Autodesk Fusion 360 part; units mm, degrees
note: some values were not read from the file. Chosen so that the rebuilt part matches the saved one: which bodies a step acts on. Set by a fixed rule: which sketch regions a step uses.
(part 5 of 6)
sketch "Sketch100" plane through (0, 0, 40) normal (0, 0, 1) x (-1, 0, 0)
  line L0 (-66.1667, -42.5926) -> (-61.6667, -42.5926)
  line L1 (-61.6667, -42.5926) -> (-61.6667, -61.6667)
  line L2 (-61.6667, -61.6667) -> (-42.5926, -61.6667)
  line L3 (-42.5926, -61.6667) -> (-42.5926, -66.1667)
  line L4 (-42.5926, -66.1667) -> (-24.0741, -66.1667)
  line L5 (-24.0741, -66.1667) -> (-24.0741, -61.6667)
  line L6 (-24.0741, -61.6667) -> (-5, -61.6667)
  line L7 (-5, -61.6667) -> (-5, -42.5926)
  line L8 (-5, -42.5926) -> (-0.5, -42.5926)
  line L9 (-0.5, -42.5926) -> (-0.5, -24.0741)
  line L10 (-0.5, -24.0741) -> (-5, -24.0741)
  line L11 (-5, -24.0741) -> (-5, -5)
  line L12 (-5, -5) -> (-24.0741, -5)
  line L13 (-24.0741, -5) -> (-24.0741, -0.5)
  line L14 (-24.0741, -0.5) -> (-42.5926, -0.5)
  line L15 (-42.5926, -0.5) -> (-42.5926, -5)
  line L16 (-42.5926, -5) -> (-61.6667, -5)
  line L17 (-61.6667, -5) -> (-61.6667, -24.0741)
  line L18 (-61.6667, -24.0741) -> (-66.1667, -24.0741)
  line L19 (-66.1667, -24.0741) -> (-66.1667, -42.5926)
  line L20 (-20.9586, -20.9586) -> (-18.6369, -23.2802)
  line L21 (-20.9586, -20.9586) -> (-23.2802, -18.6369)
  line L22 (-18.6369, -23.2802) -> (-28.69, -33.3333)
  line L23 (-18.6369, -43.3864) -> (-28.69, -33.3333)
  line L24 (-33.3333, -37.9767) -> (-43.3864, -48.0298)
  line L25 (-33.3333, -28.69) -> (-43.3864, -18.6369)
  line L26 (-20.9586, -45.7081) -> (-23.2802, -48.0298)
  line L27 (-20.9586, -45.7081) -> (-18.6369, -43.3864)
  line L28 (-23.2802, -18.6369) -> (-33.3333, -28.69)
  line L29 (-48.0298, -43.3864) -> (-37.9767, -33.3333)
  line L30 (-45.7081, -20.9586) -> (-48.0298, -23.2802)
  line L31 (-48.0298, -23.2802) -> (-37.9767, -33.3333)
  line L32 (-43.3864, -18.6369) -> (-45.7081, -20.9586)
  line L33 (-43.3864, -48.0298) -> (-45.7081, -45.7081)
  line L34 (-45.7081, -45.7081) -> (-48.0298, -43.3864)
  line L35 (-23.2802, -48.0298) -> (-33.3333, -37.9767)
  dimension "d733" = 3.2833
  dimension "d734" = 3.2833
  dimension "d735" = 14.2173
  dimension "d736" = 14.2173
  dimension "d737" = 3.2833
  dimension "d738" = 3.2833
  dimension "d739" = 28.19
  constraint perpendicular L26 L35
  constraint perpendicular L24 L35
  constraint perpendicular L29 L34
  constraint perpendicular L23 L27
  measures "d733" distance of L26.end L26.start
  measures "d734" distance of L26.start L23.start
  measures "d735" distance of L26.end L24.start
  measures "d736" distance of L24.start L24.end
  measures "d737" distance of L33.end L24.end
  measures "d738" distance of L33.end L29.start
  measures "d739" distance of L19 L29.end
extrude "Extrude61" cut sketch "Sketch93" sketch "Sketch95" sketch "Sketch97" sketch "Sketch100" sketch "Sketch96" against normal blind 4 contours L20 L21 L22 L23 L24 L25 L26 L27 L28 L29 L30 L31 L32 L33 L34 L35 of sketch 2 contours L20 L21 L22 L23 L24 L25 L26 L27 L28 L29 L30 L31 L32 L33 L34 L35 of sketch 3 contours L20 L21 L22 L23 L24 L25 L26 L27 L28 L29 L30 L31 L32 L33 L34 L35 of sketch 4 contours L20 L21 L22 L23 L24 L25 L26 L27 L28 L29 L30 L31 L32 L33 L34 L35 of sketch 5 contours L20 L21 L22 L23 L24 L25 L26 L27 L28 L29 L30 L31 L32 L33 L34 L35 bodies 13 14 15 17 18
move_body "Align1" bodies 4 to x (-0.707107, -0.707107, 0) y (0, 0, 1) z (-0.707107, 0.707107, 0) at (170.1564, 166.6217, -160)
move_body "Align2" bodies 3 to x (0, 0, 1) y (0, 1, 0) z (-1, 0, 0) at (220, 0, -160)
move_body "Align3" bodies 1 to x (0, 0, -1) y (-1, 0, 0) z (0, 1, 0) at (228.3333, 70.7407, 40)
move_body "Align4" bodies 10 to x (1, 0, 0) y (0, 0, 1) z (0, -1, 0) at (0, 110.6667, -30.6667)
move_body "Align5" bodies 11 to x (1, 0, 0) y (0, 0, 1) z (0, -1, 0) at (0, 149.3333, -97.3333)
move_body "Align6" bodies 12 to x (1, 0, 0) y (0, 0, 1) z (0, -1, 0) at (0, 133.3333, -95.3333)
move_body "Align7" bodies 5 to x (0, 0, -1) y (0, 1, 0) z (1, 0, 0) at (62.6667, 0, 100.6667)
move_body "Align8" bodies 6 to x (0, 0, 1) y (0, 1, 0) z (-1, 0, 0) at (112, -96, -28.6667)
move_body "Align9" bodies 7 to x (0, 0, -1) y (-1, 0, 0) z (0, 1, 0) at (296, 88, 167.3333)
move_body "Align10" bodies 8 to x (0, 0, -1) y (-1, 0, 0) z (0, 1, 0) at (296, 88, 171.3333)
move_body "Align11" bodies 9 to x (0, 1, 0) y (0, 0, 1) z (1, 0, 0) at (88, 96, -28.6667)
move_body "Align12" bodies 2 to x (1, 0, 0) y (0, 0, 1) z (0, -1, 0) at (0, 24, 34)
move_body "Move1" bodies 1 to x (1, 0, 0) y (0, 1, 0) z (0, 0, 1) at (-301.8229, -79.1371, 0)
move_body "Move2" bodies 2 to x (1, 0, 0) y (0, 1, 0) z (0, 0, 1) at (-268.0592, -55.8986, 0)
move_body "Move3" bodies 3 to x (1, 0, 0) y (0, 1, 0) z (0, 0, 1) at (-506.8987, -87.6592, 0)
move_body "Move4" bodies 4 to x (0.707107, 0.707107, 0) y (-0.707107, 0.707107, 0) z (0, 0, 1) at (-289.2034, -339.6643, 0)
move_body "Move5" bodies 5 to x (1, 0, 0) y (0, 1, 0) z (0, 0, 1) at (-316.3353, -293.4677, 0)
move_body "Move6" bodies 6 to x (1, 0, 0) y (0, 1, 0) z (0, 0, 1) at (-257.8958, -196.9155, 0)
move_body "Move7" bodies 7 to x (1, 0, 0) y (0, 1, 0) z (0, 0, 1) at (-204.5381, -362.0705, 0)
move_body "Move8" bodies 8 to x (1, 0, 0) y (0, 1, 0) z (0, 0, 1) at (-203.2676, -302.3606, 0)
move_body "Move9" bodies 9 to x (1, 0, 0) y (0, 1, 0) z (0, 0, 1) at (-485.6051, -398.4452, 0)
move_body "Move10" bodies 10 to x (1, 0, 0) y (0, 1, 0) z (0, 0, 1) at (-105.1453, -228.2759, 0)
move_body "Move11" bodies 11 to x (1, 0, 0) y (0, 1, 0) z (0, 0, 1) at (-55.3396, -206.1401, 0)
move_body "Move12" bodies 12 to x (1, 0, 0) y (0, 1, 0) z (0, 0, 1) at (-264.2467, -44.2717, 0)
move_body "Move13" bodies 13 to x (1, 0, 0) y (0, 1, 0) z (0, 0, 1) at (-52.5726, -34.5873, 0)
move_body "Move14" bodies 14 to x (1, 0, 0) y (0, 1, 0) z (0, 0, 1) at (-35.9707, -35.9707, 0)
move_body "Move15" bodies 15 to x (1, 0, 0) y (0, 1, 0) z (0, 0, 1) at (-13.8349, -40.1212, 0)
move_body "Move16" bodies 16 to x (1, 0, 0) y (0, 1, 0) z (0, 0, 1) at (-38.7377, -22.1358, 0)
move_body "Move17" bodies 17 to x (1, 0, 0) y (0, 1, 0) z (0, 0, 1) at (-24.9028, -20.7524, 0)
move_body "Move18" [suppressed]
move_body "Move19" [suppressed]
move_body "Move20" [suppressed]
move_body "Move21" [suppressed]
sketch "Sketch101" plane through (0, 0, 0) normal (0, 0, 1) x (1, 0, 0)
  circle A0 centre (-33.9394, 156.9822) radius 16.4167
  line L0 (-1.1061, 166.2415) -> (-5.6061, 166.2415)
  line L1 (-5.6061, 166.2415) -> (-5.6061, 185.3156)
  line L2 (-5.6061, 185.3156) -> (-24.6802, 185.3156)
  line L3 (-24.6802, 185.3156) -> (-24.6802, 189.8156)
  line L4 (-24.6802, 189.8156) -> (-43.1987, 189.8156)
  line L5 (-43.1987, 189.8156) -> (-43.1987, 185.3156)
  line L6 (-43.1987, 185.3156) -> (-62.2728, 185.3156)
  line L7 (-62.2728, 185.3156) -> (-62.2728, 166.2415)
  line L8 (-62.2728, 166.2415) -> (-66.7728, 166.2415)
  line L9 (-66.7728, 166.2415) -> (-66.7728, 147.723)
  line L10 (-66.7728, 147.723) -> (-62.2728, 147.723)
  line L11 (-62.2728, 147.723) -> (-62.2728, 128.6489)
  line L12 (-62.2728, 128.6489) -> (-43.1987, 128.6489)
  line L13 (-43.1987, 128.6489) -> (-43.1987, 124.1489)
  line L14 (-43.1987, 124.1489) -> (-24.6802, 124.1489)
  line L15 (-24.6802, 124.1489) -> (-24.6802, 128.6489)
  line L16 (-24.6802, 128.6489) -> (-5.6061, 128.6489)
  line L17 (-5.6061, 128.6489) -> (-5.6061, 147.723)
  line L18 (-5.6061, 147.723) -> (-1.1061, 147.723)
  line L19 (-1.1061, 147.723) -> (-1.1061, 166.2415)
  circle A1 centre (-128.2759, 137.6134) radius 16.4167
  line L20 (-161.1092, 128.3541) -> (-156.6092, 128.3541)
  line L21 (-156.6092, 128.3541) -> (-156.6092, 109.28)
  line L22 (-156.6092, 109.28) -> (-137.5352, 109.28)
  line L23 (-137.5352, 109.28) -> (-137.5352, 104.78)
  line L24 (-137.5352, 104.78) -> (-119.0166, 104.78)
  line L25 (-119.0166, 104.78) -> (-119.0166, 109.28)
  line L26 (-119.0166, 109.28) -> (-99.9426, 109.28)
  line L27 (-99.9426, 109.28) -> (-99.9426, 128.3541)
  line L28 (-99.9426, 128.3541) -> (-95.4426, 128.3541)
  line L29 (-95.4426, 128.3541) -> (-95.4426, 146.8726)
  line L30 (-95.4426, 146.8726) -> (-99.9426, 146.8726)
  line L31 (-99.9426, 146.8726) -> (-99.9426, 165.9467)
  line L32 (-99.9426, 165.9467) -> (-119.0166, 165.9467)
  line L33 (-119.0166, 165.9467) -> (-119.0166, 170.4467)
  line L34 (-119.0166, 170.4467) -> (-137.5352, 170.4467)
  line L35 (-137.5352, 170.4467) -> (-137.5352, 165.9467)
  line L36 (-137.5352, 165.9467) -> (-156.6092, 165.9467)
  line L37 (-156.6092, 165.9467) -> (-156.6092, 146.8726)
  line L38 (-156.6092, 146.8726) -> (-161.1092, 146.8726)
  line L39 (-161.1092, 146.8726) -> (-161.1092, 128.3541)
  circle A2 centre (-200.4765, 134.8464) radius 16.4167
  line L40 (-167.6432, 144.1056) -> (-172.1432, 144.1056)
  line L41 (-172.1432, 144.1056) -> (-172.1432, 163.1797)
  line L42 (-172.1432, 163.1797) -> (-191.2173, 163.1797)
  line L43 (-191.2173, 163.1797) -> (-191.2173, 167.6797)
  line L44 (-191.2173, 167.6797) -> (-209.7358, 167.6797)
  line L45 (-209.7358, 167.6797) -> (-209.7358, 163.1797)
  line L46 (-209.7358, 163.1797) -> (-228.8099, 163.1797)
  line L47 (-228.8099, 163.1797) -> (-228.8099, 144.1056)
  line L48 (-228.8099, 144.1056) -> (-233.3099, 144.1056)
  line L49 (-233.3099, 144.1056) -> (-233.3099, 125.5871)
  line L50 (-233.3099, 125.5871) -> (-228.8099, 125.5871)
  line L51 (-228.8099, 125.5871) -> (-228.8099, 106.5131)
  line L52 (-228.8099, 106.5131) -> (-209.7358, 106.5131)
  line L53 (-209.7358, 106.5131) -> (-209.7358, 102.0131)
  line L54 (-209.7358, 102.0131) -> (-191.2173, 102.0131)
  line L55 (-191.2173, 102.0131) -> (-191.2173, 106.5131)
  line L56 (-191.2173, 106.5131) -> (-172.1432, 106.5131)
  line L57 (-172.1432, 106.5131) -> (-172.1432, 125.5871)
  line L58 (-172.1432, 125.5871) -> (-167.6432, 125.5871)
  line L59 (-167.6432, 125.5871) -> (-167.6432, 144.1056)
  line L60 (-326.8987, 90.1186) -> (-322.8987, 90.1186)
  line L61 (-322.8987, 90.1186) -> (-322.8987, 67.8964)
  line L62 (-322.8987, 67.8964) -> (-326.8987, 67.8964)
  line L63 (-326.8987, 67.8964) -> (-326.8987, 23.4519)
  line L64 (-326.8987, 23.4519) -> (-322.8987, 23.4519)
  line L65 (-322.8987, 23.4519) -> (-322.8987, 1.2297)
  line L66 (-322.8987, 1.2297) -> (-326.8987, 1.2297)
  line L67 (-326.8987, 1.2297) -> (-326.8987, -43.2147)
  line L68 (-326.8987, -43.2147) -> (-322.8987, -43.2147)
  line L69 (-322.8987, -43.2147) -> (-322.8987, -65.4369)
  line L70 (-322.8987, -65.4369) -> (-326.8987, -65.4369)
  line L71 (-326.8987, -65.4369) -> (-326.8987, -87.6592)
  line L72 (-326.8987, -87.6592) -> (-318.8987, -87.6592)
  line L73 (-318.8987, -87.6592) -> (-318.8987, -83.6592)
  line L74 (-318.8987, -83.6592) -> (-310.8987, -83.6592)
  line L75 (-310.8987, -83.6592) -> (-310.8987, -87.6592)
  line L76 (-310.8987, -87.6592) -> (-302.8987, -87.6592)
  line L77 (-302.8987, -87.6592) -> (-302.8987, -83.6592)
  line L78 (-302.8987, -83.6592) -> (-294.8987, -83.6592)
  line L79 (-294.8987, -83.6592) -> (-294.8987, -87.6592)
  line L80 (-294.8987, -87.6592) -> (-286.8987, -87.6592)
  line L81 (-286.8987, -87.6592) -> (-286.8987, 112.3408)
  line L82 (-286.8987, 112.3408) -> (-294.8987, 112.3408)
  line L83 (-294.8987, 112.3408) -> (-294.8987, 108.3408)
  line L84 (-294.8987, 108.3408) -> (-302.8987, 108.3408)
  line L85 (-302.8987, 108.3408) -> (-302.8987, 112.3408)
  line L86 (-302.8987, 112.3408) -> (-310.8987, 112.3408)
  line L87 (-310.8987, 112.3408) -> (-310.8987, 108.3408)
  line L88 (-310.8987, 108.3408) -> (-318.8987, 108.3408)
  line L89 (-318.8987, 108.3408) -> (-318.8987, 112.3408)
  line L90 (-318.8987, 112.3408) -> (-326.8987, 112.3408)
  line L91 (-326.8987, 112.3408) -> (-326.8987, 90.1186)
  line L92 (-314.8987, 49.6742) -> (-298.8987, 49.6742)
  line L93 (-298.8987, 49.6742) -> (-298.8987, 41.6742)
  line L94 (-298.8987, 41.6742) -> (-314.8987, 41.6742)
  line L95 (-314.8987, 41.6742) -> (-314.8987, 49.6742)
  line L96 (-314.8987, -16.9925) -> (-298.8987, -16.9925)
  line L97 (-298.8987, -16.9925) -> (-298.8987, -24.9925)
  line L98 (-298.8987, -24.9925) -> (-314.8987, -24.9925)
  line L99 (-314.8987, -24.9925) -> (-314.8987, -16.9925)
  line L100 (-86.4689, 53.0616) -> (-86.4689, 49.0616)
  line L101 (-86.4689, 49.0616) -> (-68.2467, 49.0616)
  line L102 (-68.2467, 49.0616) -> (-68.2467, 61.0616)
  line L103 (-68.2467, 61.0616) -> (-64.2467, 61.0616)
  line L104 (-64.2467, 61.0616) -> (-64.2467, 77.0616)
  line L105 (-64.2467, 77.0616) -> (-68.2467, 77.0616)
  line L106 (-68.2467, 77.0616) -> (-68.2467, 89.0616)
  line L107 (-68.2467, 89.0616) -> (-260.2467, 89.0616)
  line L108 (-260.2467, 89.0616) -> (-260.2467, 77.0616)
  line L109 (-260.2467, 77.0616) -> (-264.2467, 77.0616)
  line L110 (-264.2467, 77.0616) -> (-264.2467, 61.0616)
  line L111 (-264.2467, 61.0616) -> (-260.2467, 61.0616)
  line L112 (-260.2467, 61.0616) -> (-260.2467, 49.0616)
  line L113 (-260.2467, 49.0616) -> (-242.0244, 49.0616)
  line L114 (-242.0244, 49.0616) -> (-242.0244, 53.0616)
  line L115 (-242.0244, 53.0616) -> (-219.8022, 53.0616)
  line L116 (-219.8022, 53.0616) -> (-219.8022, 49.0616)
  line L117 (-219.8022, 49.0616) -> (-201.58, 49.0616)
  line L118 (-201.58, 49.0616) -> (-201.58, 69.0616)
  line L119 (-201.58, 69.0616) -> (-193.58, 69.0616)
  line L120 (-193.58, 69.0616) -> (-193.58, 49.0616)
  line L121 (-193.58, 49.0616) -> (-175.3578, 49.0616)
  line L122 (-175.3578, 49.0616) -> (-175.3578, 53.0616)
  line L123 (-175.3578, 53.0616) -> (-153.1355, 53.0616)
  line L124 (-153.1355, 53.0616) -> (-153.1355, 49.0616)
  line L125 (-153.1355, 49.0616) -> (-134.9133, 49.0616)
  line L126 (-134.9133, 49.0616) -> (-134.9133, 69.0616)
  line L127 (-134.9133, 69.0616) -> (-126.9133, 69.0616)
  line L128 (-126.9133, 69.0616) -> (-126.9133, 49.0616)
  line L129 (-126.9133, 49.0616) -> (-108.6911, 49.0616)
  line L130 (-108.6911, 49.0616) -> (-108.6911, 53.0616)
  line L131 (-108.6911, 53.0616) -> (-86.4689, 53.0616)
  circle A3 centre (-5.4044, 77.8642) radius 16.4167
  line L132 (27.4289, 87.1234) -> (22.9289, 87.1234)
  line L133 (22.9289, 87.1234) -> (22.9289, 106.1975)
  line L134 (22.9289, 106.1975) -> (3.8549, 106.1975)
  line L135 (3.8549, 106.1975) -> (3.8549, 110.6975)
  line L136 (3.8549, 110.6975) -> (-14.6637, 110.6975)
  line L137 (-14.6637, 110.6975) -> (-14.6637, 106.1975)
  line L138 (-14.6637, 106.1975) -> (-33.7377, 106.1975)
  line L139 (-33.7377, 106.1975) -> (-33.7377, 87.1234)
  line L140 (-33.7377, 87.1234) -> (-38.2377, 87.1234)
  line L141 (-38.2377, 87.1234) -> (-38.2377, 68.6049)
  line L142 (-38.2377, 68.6049) -> (-33.7377, 68.6049)
  line L143 (-33.7377, 68.6049) -> (-33.7377, 49.5308)
  line L144 (-33.7377, 49.5308) -> (-14.6637, 49.5308)
  line L145 (-14.6637, 49.5308) -> (-14.6637, 45.0308)
  line L146 (-14.6637, 45.0308) -> (3.8549, 45.0308)
  line L147 (3.8549, 45.0308) -> (3.8549, 49.5308)
  line L148 (3.8549, 49.5308) -> (22.9289, 49.5308)
  line L149 (22.9289, 49.5308) -> (22.9289, 68.6049)
  line L150 (22.9289, 68.6049) -> (27.4289, 68.6049)
  line L151 (27.4289, 68.6049) -> (27.4289, 87.1234)
  line L152 (162.8849, -21.4843) -> (152.8318, -11.4312)
  line L153 (152.8318, -11.4312) -> (142.7786, -21.4843)
  line L154 (142.7786, -21.4843) -> (138.1353, -16.841)
  line L155 (138.1353, -16.841) -> (148.1884, -6.7879)
  line L156 (148.1884, -6.7879) -> (138.1353, 3.2652)
  line L157 (138.1353, 3.2652) -> (142.7786, 7.9086)
  line L158 (142.7786, 7.9086) -> (152.8318, -2.1446)
  line L159 (152.8318, -2.1446) -> (162.8849, 7.9086)
  line L160 (162.8849, 7.9086) -> (167.5282, 3.2652)
  line L161 (167.5282, 3.2652) -> (157.4751, -6.7879)
  line L162 (157.4751, -6.7879) -> (167.5282, -16.841)
  line L163 (167.5282, -16.841) -> (162.8849, -21.4843)
  line L164 (143.5725, 26.0454) -> (143.5725, 21.5454)
  line L165 (143.5725, 21.5454) -> (124.4984, 21.5454)
  line L166 (124.4984, 21.5454) -> (124.4984, 2.4714)
  line L167 (124.4984, 2.4714) -> (119.9984, 2.4714)
  line L168 (119.9984, 2.4714) -> (119.9984, -16.0471)
  line L169 (119.9984, -16.0471) -> (124.4984, -16.0471)
  line L170 (124.4984, -16.0471) -> (124.4984, -35.1212)
  line L171 (124.4984, -35.1212) -> (143.5725, -35.1212)
  line L172 (143.5725, -35.1212) -> (143.5725, -39.6212)
  line L173 (143.5725, -39.6212) -> (162.091, -39.6212)
  line L174 (162.091, -39.6212) -> (162.091, -35.1212)
  line L175 (162.091, -35.1212) -> (181.1651, -35.1212)
  line L176 (181.1651, -35.1212) -> (181.1651, -16.0471)
  line L177 (181.1651, -16.0471) -> (185.6651, -16.0471)
  line L178 (185.6651, -16.0471) -> (185.6651, 2.4714)
  line L179 (185.6651, 2.4714) -> (181.1651, 2.4714)
  line L180 (181.1651, 2.4714) -> (181.1651, 21.5454)
  line L181 (181.1651, 21.5454) -> (162.091, 21.5454)
  line L182 (162.091, 21.5454) -> (162.091, 26.0454)
  line L183 (162.091, 26.0454) -> (143.5725, 26.0454)
  line L184 (64.0293, -7.2808) -> (53.9761, -17.3339)
  line L185 (53.9761, -17.3339) -> (49.3328, -12.6905)
  line L186 (49.3328, -12.6905) -> (59.3859, -2.6374)
  line L187 (59.3859, -2.6374) -> (49.3328, 7.4157)
  line L188 (49.3328, 7.4157) -> (53.9761, 12.059)
  line L189 (53.9761, 12.059) -> (64.0293, 2.0059)
  line L190 (64.0293, 2.0059) -> (74.0824, 12.059)
  line L191 (74.0824, 12.059) -> (78.7257, 7.4157)
  line L192 (78.7257, 7.4157) -> (68.6726, -2.6374)
  line L193 (68.6726, -2.6374) -> (78.7257, -12.6905)
  line L194 (78.7257, -12.6905) -> (74.0824, -17.3339)
  line L195 (74.0824, -17.3339) -> (64.0293, -7.2808)
  line L196 (31.1959, -11.8967) -> (35.6959, -11.8967)
  line L197 (35.6959, -11.8967) -> (35.6959, -30.9707)
  line L198 (35.6959, -30.9707) -> (54.77, -30.9707)
  line L199 (54.77, -30.9707) -> (54.77, -35.4707)
  line L200 (54.77, -35.4707) -> (73.2885, -35.4707)
  line L201 (73.2885, -35.4707) -> (73.2885, -30.9707)
  line L202 (73.2885, -30.9707) -> (92.3626, -30.9707)
  line L203 (92.3626, -30.9707) -> (92.3626, -11.8967)
  line L204 (92.3626, -11.8967) -> (96.8626, -11.8967)
  line L205 (96.8626, -11.8967) -> (96.8626, 6.6218)
  line L206 (96.8626, 6.6218) -> (92.3626, 6.6218)
  line L207 (92.3626, 6.6218) -> (92.3626, 25.6959)
  line L208 (92.3626, 25.6959) -> (73.2885, 25.6959)
  line L209 (73.2885, 25.6959) -> (73.2885, 30.1959)
  line L210 (73.2885, 30.1959) -> (54.77, 30.1959)
  line L211 (54.77, 30.1959) -> (54.77, 25.6959)
  line L212 (54.77, 25.6959) -> (35.6959, 25.6959)
  line L213 (35.6959, 25.6959) -> (35.6959, 6.6218)
  line L214 (35.6959, 6.6218) -> (31.1959, 6.6218)
  line L215 (31.1959, 6.6218) -> (31.1959, -11.8967)
  line L216 (-23.8826, -1.2539) -> (-33.9357, 8.7992)
  line L217 (-33.9357, 8.7992) -> (-29.2924, 13.4425)
  line L218 (-29.2924, 13.4425) -> (-19.2393, 3.3894)
  line L219 (-19.2393, 3.3894) -> (-9.1862, 13.4425)
  line L220 (-9.1862, 13.4425) -> (-4.5429, 8.7992)
  line L221 (-4.5429, 8.7992) -> (-14.596, -1.2539)
  line L222 (-14.596, -1.2539) -> (-4.5429, -11.307)
  line L223 (-4.5429, -11.307) -> (-9.1862, -15.9504)
  line L224 (-9.1862, -15.9504) -> (-19.2393, -5.8973)
  line L225 (-19.2393, -5.8973) -> (-29.2924, -15.9504)
  line L226 (-29.2924, -15.9504) -> (-33.9357, -11.307)
  line L227 (-33.9357, -11.307) -> (-23.8826, -1.2539)
  line L228 (13.594, 8.0053) -> (9.094, 8.0053)
  line L229 (9.094, 8.0053) -> (9.094, 27.0794)
  line L230 (9.094, 27.0794) -> (-9.98, 27.0794)
  line L231 (-9.98, 27.0794) -> (-9.98, 31.5794)
  line L232 (-9.98, 31.5794) -> (-28.4986, 31.5794)
  line L233 (-28.4986, 31.5794) -> (-28.4986, 27.0794)
  line L234 (-28.4986, 27.0794) -> (-47.5726, 27.0794)
  line L235 (-47.5726, 27.0794) -> (-47.5726, 8.0053)
  line L236 (-47.5726, 8.0053) -> (-52.0726, 8.0053)
  line L237 (-52.0726, 8.0053) -> (-52.0726, -10.5132)
  line L238 (-52.0726, -10.5132) -> (-47.5726, -10.5132)
  line L239 (-47.5726, -10.5132) -> (-47.5726, -29.5873)
  line L240 (-47.5726, -29.5873) -> (-28.4986, -29.5873)
  line L241 (-28.4986, -29.5873) -> (-28.4986, -34.0873)
  line L242 (-28.4986, -34.0873) -> (-9.98, -34.0873)
  line L243 (-9.98, -34.0873) -> (-9.98, -29.5873)
  line L244 (-9.98, -29.5873) -> (9.094, -29.5873)
  line L245 (9.094, -29.5873) -> (9.094, -10.5132)
  line L246 (9.094, -10.5132) -> (13.594, -10.5132)
  line L247 (13.594, -10.5132) -> (13.594, 8.0053)
  line L248 (122.4382, -92.8067) -> (122.4382, -96.8067)
  line L249 (122.4382, -96.8067) -> (140.6604, -96.8067)
  line L250 (140.6604, -96.8067) -> (140.6604, -84.8067)
  line L251 (140.6604, -84.8067) -> (144.6604, -84.8067)
  line L252 (144.6604, -84.8067) -> (144.6604, -68.8067)
  line L253 (144.6604, -68.8067) -> (140.6604, -68.8067)
  line L254 (140.6604, -68.8067) -> (140.6604, -56.8067)
  line L255 (140.6604, -56.8067) -> (-51.3396, -56.8067)
  line L256 (-51.3396, -56.8067) -> (-51.3396, -68.8067)
  line L257 (-51.3396, -68.8067) -> (-55.3396, -68.8067)
  line L258 (-55.3396, -68.8067) -> (-55.3396, -84.8067)
  line L259 (-55.3396, -84.8067) -> (-51.3396, -84.8067)
  line L260 (-51.3396, -84.8067) -> (-51.3396, -96.8067)
  line L261 (-51.3396, -96.8067) -> (-33.1174, -96.8067)
  line L262 (-33.1174, -96.8067) -> (-33.1174, -92.8067)
  line L263 (-33.1174, -92.8067) -> (-10.8952, -92.8067)
  line L264 (-10.8952, -92.8067) -> (-10.8952, -96.8067)
  line L265 (-10.8952, -96.8067) -> (7.3271, -96.8067)
  line L266 (7.3271, -96.8067) -> (7.3271, -76.8067)
  line L267 (7.3271, -76.8067) -> (15.3271, -76.8067)
  line L268 (15.3271, -76.8067) -> (15.3271, -96.8067)
  line L269 (15.3271, -96.8067) -> (33.5493, -96.8067)
  line L270 (33.5493, -96.8067) -> (33.5493, -92.8067)
  line L271 (33.5493, -92.8067) -> (55.7715, -92.8067)
  line L272 (55.7715, -92.8067) -> (55.7715, -96.8067)
  line L273 (55.7715, -96.8067) -> (73.9937, -96.8067)
  line L274 (73.9937, -96.8067) -> (73.9937, -76.8067)
  line L275 (73.9937, -76.8067) -> (81.9937, -76.8067)
  line L276 (81.9937, -76.8067) -> (81.9937, -96.8067)
  line L277 (81.9937, -96.8067) -> (100.2159, -96.8067)
  line L278 (100.2159, -96.8067) -> (100.2159, -92.8067)
  line L279 (100.2159, -92.8067) -> (122.4382, -92.8067)
  line L280 (-90.2814, -67.8986) -> (-90.2814, -71.8986)
  line L281 (-90.2814, -71.8986) -> (-72.0592, -71.8986)
  line L282 (-72.0592, -71.8986) -> (-72.0592, -63.8986)
  line L283 (-72.0592, -63.8986) -> (-68.0592, -63.8986)
  line L284 (-68.0592, -63.8986) -> (-68.0592, -55.8986)
  line L285 (-68.0592, -55.8986) -> (-72.0592, -55.8986)
  line L286 (-72.0592, -55.8986) -> (-72.0592, -47.8986)
  line L287 (-72.0592, -47.8986) -> (-68.0592, -47.8986)
  line L288 (-68.0592, -47.8986) -> (-68.0592, -39.8986)
  line L289 (-68.0592, -39.8986) -> (-72.0592, -39.8986)
  line L290 (-72.0592, -39.8986) -> (-72.0592, -31.8986)
  line L291 (-72.0592, -31.8986) -> (-264.0592, -31.8986)
  line L292 (-264.0592, -31.8986) -> (-264.0592, -39.8986)
  line L293 (-264.0592, -39.8986) -> (-268.0592, -39.8986)
  line L294 (-268.0592, -39.8986) -> (-268.0592, -47.8986)
  line L295 (-268.0592, -47.8986) -> (-264.0592, -47.8986)
  line L296 (-264.0592, -47.8986) -> (-264.0592, -55.8986)
  line L297 (-264.0592, -55.8986) -> (-268.0592, -55.8986)
  line L298 (-268.0592, -55.8986) -> (-268.0592, -63.8986)
  line L299 (-268.0592, -63.8986) -> (-264.0592, -63.8986)
  line L300 (-264.0592, -63.8986) -> (-264.0592, -71.8986)
  line L301 (-264.0592, -71.8986) -> (-245.837, -71.8986)
  line L302 (-245.837, -71.8986) -> (-245.837, -67.8986)
  line L303 (-245.837, -67.8986) -> (-223.6148, -67.8986)
  line L304 (-223.6148, -67.8986) -> (-223.6148, -71.8986)
  line L305 (-223.6148, -71.8986) -> (-179.1703, -71.8986)
  line L306 (-179.1703, -71.8986) -> (-179.1703, -67.8986)
  line L307 (-179.1703, -67.8986) -> (-156.9481, -67.8986)
  line L308 (-156.9481, -67.8986) -> (-156.9481, -71.8986)
  line L309 (-156.9481, -71.8986) -> (-112.5036, -71.8986)
  line L310 (-112.5036, -71.8986) -> (-112.5036, -67.8986)
  line L311 (-112.5036, -67.8986) -> (-90.2814, -67.8986)
  line L312 (-130.7259, -43.8986) -> (-130.7259, -59.8986)
  line L313 (-130.7259, -59.8986) -> (-138.7259, -59.8986)
  line L314 (-138.7259, -59.8986) -> (-138.7259, -43.8986)
  line L315 (-138.7259, -43.8986) -> (-130.7259, -43.8986)
  line L316 (-197.3925, -43.8986) -> (-197.3925, -59.8986)
  line L317 (-197.3925, -59.8986) -> (-205.3925, -59.8986)
  line L318 (-205.3925, -59.8986) -> (-205.3925, -43.8986)
  line L319 (-205.3925, -43.8986) -> (-197.3925, -43.8986)
  line L320 (-117.934, 27.6036) -> (-117.934, 31.6036)
  line L321 (-117.934, 31.6036) -> (-162.3784, 31.6036)
  line L322 (-162.3784, 31.6036) -> (-162.3784, 27.6036)
  line L323 (-162.3784, 27.6036) -> (-184.6007, 27.6036)
  line L324 (-184.6007, 27.6036) -> (-184.6007, 31.6036)
  line L325 (-184.6007, 31.6036) -> (-229.0451, 31.6036)
  line L326 (-229.0451, 31.6036) -> (-229.0451, 27.6036)
  line L327 (-229.0451, 27.6036) -> (-251.2673, 27.6036)
  line L328 (-251.2673, 27.6036) -> (-251.2673, 31.6036)
  line L329 (-251.2673, 31.6036) -> (-273.4895, 31.6036)
  line L330 (-273.4895, 31.6036) -> (-273.4895, 23.6036)
  line L331 (-273.4895, 23.6036) -> (-269.4895, 23.6036)
  line L332 (-269.4895, 23.6036) -> (-269.4895, 15.6036)
  line L333 (-269.4895, 15.6036) -> (-273.4895, 15.6036)
  line L334 (-273.4895, 15.6036) -> (-273.4895, 7.6036)
  line L335 (-273.4895, 7.6036) -> (-269.4895, 7.6036)
  line L336 (-269.4895, 7.6036) -> (-269.4895, -0.3964)
  line L337 (-269.4895, -0.3964) -> (-273.4895, -0.3964)
  line L338 (-273.4895, -0.3964) -> (-273.4895, -8.3964)
  line L339 (-273.4895, -8.3964) -> (-73.4895, -8.3964)
  line L340 (-73.4895, -8.3964) -> (-73.4895, -0.3964)
  line L341 (-73.4895, -0.3964) -> (-77.4895, -0.3964)
  line L342 (-77.4895, -0.3964) -> (-77.4895, 7.6036)
  line L343 (-77.4895, 7.6036) -> (-73.4895, 7.6036)
  line L344 (-73.4895, 7.6036) -> (-73.4895, 15.6036)
  line L345 (-73.4895, 15.6036) -> (-77.4895, 15.6036)
  line L346 (-77.4895, 15.6036) -> (-77.4895, 23.6036)
  line L347 (-77.4895, 23.6036) -> (-73.4895, 23.6036)
  line L348 (-73.4895, 23.6036) -> (-73.4895, 31.6036)
  line L349 (-73.4895, 31.6036) -> (-95.7118, 31.6036)
  line L350 (-95.7118, 31.6036) -> (-95.7118, 27.6036)
  line L351 (-95.7118, 27.6036) -> (-117.934, 27.6036)
  line L352 (-136.1562, 19.6036) -> (-136.1562, 3.6036)
  line L353 (-136.1562, 3.6036) -> (-144.1562, 3.6036)
  line L354 (-144.1562, 3.6036) -> (-144.1562, 19.6036)
  line L355 (-144.1562, 19.6036) -> (-136.1562, 19.6036)
  line L356 (-202.8229, 19.6036) -> (-202.8229, 3.6036)
  line L357 (-202.8229, 3.6036) -> (-210.8229, 3.6036)
  line L358 (-210.8229, 3.6036) -> (-210.8229, 19.6036)
  line L359 (-210.8229, 19.6036) -> (-202.8229, 19.6036)
  line L360 (-181.8958, -137.36) -> (-185.8958, -137.36)
  line L361 (-185.8958, -137.36) -> (-185.8958, -181.8044)
  line L362 (-185.8958, -181.8044) -> (-181.8958, -181.8044)
  line L363 (-181.8958, -181.8044) -> (-181.8958, -204.0266)
  line L364 (-181.8958, -204.0266) -> (-185.8958, -204.0266)
  line L365 (-185.8958, -204.0266) -> (-185.8958, -248.4711)
  line L366 (-185.8958, -248.4711) -> (-181.8958, -248.4711)
  line L367 (-181.8958, -248.4711) -> (-181.8958, -270.6933)
  line L368 (-181.8958, -270.6933) -> (-185.8958, -270.6933)
  line L369 (-185.8958, -270.6933) -> (-185.8958, -288.9155)
  line L370 (-185.8958, -288.9155) -> (-173.8958, -288.9155)
  line L371 (-173.8958, -288.9155) -> (-173.8958, -292.9155)
  line L372 (-173.8958, -292.9155) -> (-157.8958, -292.9155)
  line L373 (-157.8958, -292.9155) -> (-157.8958, -288.9155)
  line L374 (-157.8958, -288.9155) -> (-145.8958, -288.9155)
  line L375 (-145.8958, -288.9155) -> (-145.8958, -230.2489)
  line L376 (-145.8958, -230.2489) -> (-165.8958, -230.2489)
  line L377 (-165.8958, -230.2489) -> (-165.8958, -222.2489)
  line L378 (-165.8958, -222.2489) -> (-145.8958, -222.2489)
  line L379 (-145.8958, -222.2489) -> (-145.8958, -163.5822)
  line L380 (-145.8958, -163.5822) -> (-165.8958, -163.5822)
  line L381 (-165.8958, -163.5822) -> (-165.8958, -155.5822)
  line L382 (-165.8958, -155.5822) -> (-145.8958, -155.5822)
  line L383 (-145.8958, -155.5822) -> (-145.8958, -96.9155)
  line L384 (-145.8958, -96.9155) -> (-157.8958, -96.9155)
  line L385 (-157.8958, -96.9155) -> (-157.8958, -92.9155)
  line L386 (-157.8958, -92.9155) -> (-173.8958, -92.9155)
  line L387 (-173.8958, -92.9155) -> (-173.8958, -96.9155)
  line L388 (-173.8958, -96.9155) -> (-185.8958, -96.9155)
  line L389 (-185.8958, -96.9155) -> (-185.8958, -115.1377)
  line L390 (-185.8958, -115.1377) -> (-181.8958, -115.1377)
  line L391 (-181.8958, -115.1377) -> (-181.8958, -137.36)
  line L392 (-213.6686, -137.9121) -> (-217.6686, -137.9121)
  line L393 (-217.6686, -137.9121) -> (-217.6686, -115.6899)
  line L394 (-217.6686, -115.6899) -> (-213.6686, -115.6899)
  line L395 (-213.6686, -115.6899) -> (-213.6686, -97.4677)
  line L396 (-213.6686, -97.4677) -> (-225.6686, -97.4677)
  line L397 (-225.6686, -97.4677) -> (-225.6686, -93.4677)
  line L398 (-225.6686, -93.4677) -> (-241.6686, -93.4677)
  line L399 (-241.6686, -93.4677) -> (-241.6686, -97.4677)
  line L400 (-241.6686, -97.4677) -> (-253.6686, -97.4677)
  line L401 (-253.6686, -97.4677) -> (-253.6686, -156.1343)
  line L402 (-253.6686, -156.1343) -> (-233.6686, -156.1343)
  line L403 (-233.6686, -156.1343) -> (-233.6686, -164.1343)
  line L404 (-233.6686, -164.1343) -> (-253.6686, -164.1343)
  line L405 (-253.6686, -164.1343) -> (-253.6686, -222.801)
  line L406 (-253.6686, -222.801) -> (-233.6686, -222.801)
  line L407 (-233.6686, -222.801) -> (-233.6686, -230.801)
  line L408 (-233.6686, -230.801) -> (-253.6686, -230.801)
  line L409 (-253.6686, -230.801) -> (-253.6686, -289.4677)
  line L410 (-253.6686, -289.4677) -> (-241.6686, -289.4677)
  line L411 (-241.6686, -289.4677) -> (-241.6686, -293.4677)
  line L412 (-241.6686, -293.4677) -> (-225.6686, -293.4677)
  line L413 (-225.6686, -293.4677) -> (-225.6686, -289.4677)
  line L414 (-225.6686, -289.4677) -> (-213.6686, -289.4677)
  line L415 (-213.6686, -289.4677) -> (-213.6686, -271.2454)
  line L416 (-213.6686, -271.2454) -> (-217.6686, -271.2454)
  line L417 (-217.6686, -271.2454) -> (-217.6686, -249.0232)
  line L418 (-217.6686, -249.0232) -> (-213.6686, -249.0232)
  line L419 (-213.6686, -249.0232) -> (-213.6686, -204.5788)
  line L420 (-213.6686, -204.5788) -> (-217.6686, -204.5788)
  line L421 (-217.6686, -204.5788) -> (-217.6686, -182.3565)
  line L422 (-217.6686, -182.3565) -> (-213.6686, -182.3565)
  line L423 (-213.6686, -182.3565) -> (-213.6686, -137.9121)
  line L424 (-322.704, -145.9707) -> (-326.704, -145.9707)
  line L425 (-326.704, -145.9707) -> (-326.704, -190.4151)
  line L426 (-326.704, -190.4151) -> (-322.704, -190.4151)
  line L427 (-322.704, -190.4151) -> (-322.704, -212.6374)
  line L428 (-322.704, -212.6374) -> (-326.704, -212.6374)
  line L429 (-326.704, -212.6374) -> (-326.704, -257.0818)
  line L430 (-326.704, -257.0818) -> (-322.704, -257.0818)
  line L431 (-322.704, -257.0818) -> (-322.704, -279.304)
  line L432 (-322.704, -279.304) -> (-326.704, -279.304)
  line L433 (-326.704, -279.304) -> (-326.704, -297.5263)
  line L434 (-326.704, -297.5263) -> (-318.704, -297.5263)
  line L435 (-318.704, -297.5263) -> (-318.704, -301.5263)
  line L436 (-318.704, -301.5263) -> (-310.704, -301.5263)
  line L437 (-310.704, -301.5263) -> (-310.704, -297.5263)
  line L438 (-310.704, -297.5263) -> (-302.704, -297.5263)
  line L439 (-302.704, -297.5263) -> (-302.704, -301.5263)
  line L440 (-302.704, -301.5263) -> (-294.704, -301.5263)
  line L441 (-294.704, -301.5263) -> (-294.704, -297.5263)
  line L442 (-294.704, -297.5263) -> (-286.704, -297.5263)
  line L443 (-286.704, -297.5263) -> (-286.704, -105.5263)
  line L444 (-286.704, -105.5263) -> (-294.704, -105.5263)
  line L445 (-294.704, -105.5263) -> (-294.704, -101.5263)
  line L446 (-294.704, -101.5263) -> (-302.704, -101.5263)
  line L447 (-302.704, -101.5263) -> (-302.704, -105.5263)
  line L448 (-302.704, -105.5263) -> (-310.704, -105.5263)
  line L449 (-310.704, -105.5263) -> (-310.704, -101.5263)
  line L450 (-310.704, -101.5263) -> (-318.704, -101.5263)
  line L451 (-318.704, -101.5263) -> (-318.704, -105.5263)
  line L452 (-318.704, -105.5263) -> (-326.704, -105.5263)
  line L453 (-326.704, -105.5263) -> (-326.704, -123.7485)
  line L454 (-326.704, -123.7485) -> (-322.704, -123.7485)
  line L455 (-322.704, -123.7485) -> (-322.704, -145.9707)
  line L456 (-314.704, -164.1929) -> (-298.704, -164.1929)
  line L457 (-298.704, -164.1929) -> (-298.704, -172.1929)
  line L458 (-298.704, -172.1929) -> (-314.704, -172.1929)
  line L459 (-314.704, -172.1929) -> (-314.704, -164.1929)
  line L460 (-314.704, -230.8596) -> (-298.704, -230.8596)
  line L461 (-298.704, -230.8596) -> (-298.704, -238.8596)
  line L462 (-298.704, -238.8596) -> (-314.704, -238.8596)
  line L463 (-314.704, -238.8596) -> (-314.704, -230.8596)
  line L464 (-361.6051, -258.0008) -> (-357.6051, -258.0008)
  line L465 (-357.6051, -258.0008) -> (-357.6051, -239.7786)
  line L466 (-357.6051, -239.7786) -> (-377.6051, -239.7786)
  line L467 (-377.6051, -239.7786) -> (-377.6051, -231.7786)
  line L468 (-377.6051, -231.7786) -> (-357.6051, -231.7786)
  line L469 (-357.6051, -231.7786) -> (-357.6051, -213.5563)
  line L470 (-357.6051, -213.5563) -> (-361.6051, -213.5563)
  line L471 (-361.6051, -213.5563) -> (-361.6051, -191.3341)
  line L472 (-361.6051, -191.3341) -> (-357.6051, -191.3341)
  line L473 (-357.6051, -191.3341) -> (-357.6051, -173.1119)
  line L474 (-357.6051, -173.1119) -> (-377.6051, -173.1119)
  line L475 (-377.6051, -173.1119) -> (-377.6051, -165.1119)
  line L476 (-377.6051, -165.1119) -> (-357.6051, -165.1119)
  line L477 (-357.6051, -165.1119) -> (-357.6051, -146.8897)
  line L478 (-357.6051, -146.8897) -> (-361.6051, -146.8897)
  line L479 (-361.6051, -146.8897) -> (-361.6051, -124.6674)
  line L480 (-361.6051, -124.6674) -> (-357.6051, -124.6674)
  line L481 (-357.6051, -124.6674) -> (-357.6051, -106.4452)
  line L482 (-357.6051, -106.4452) -> (-369.6051, -106.4452)
  line L483 (-369.6051, -106.4452) -> (-369.6051, -102.4452)
  line L484 (-369.6051, -102.4452) -> (-385.6051, -102.4452)
  line L485 (-385.6051, -102.4452) -> (-385.6051, -106.4452)
  line L486 (-385.6051, -106.4452) -> (-397.6051, -106.4452)
  line L487 (-397.6051, -106.4452) -> (-397.6051, -298.4452)
  line L488 (-397.6051, -298.4452) -> (-385.6051, -298.4452)
  line L489 (-385.6051, -298.4452) -> (-385.6051, -302.4452)
  line L490 (-385.6051, -302.4452) -> (-369.6051, -302.4452)
  line L491 (-369.6051, -302.4452) -> (-369.6051, -298.4452)
  line L492 (-369.6051, -298.4452) -> (-357.6051, -298.4452)
  line L493 (-357.6051, -298.4452) -> (-357.6051, -280.223)
  line L494 (-357.6051, -280.223) -> (-361.6051, -280.223)
  line L495 (-361.6051, -280.223) -> (-361.6051, -258.0008)
  line L496 (-82.923, -157.6092) -> (-82.923, -153.6092)
  line L497 (-82.923, -153.6092) -> (-60.7008, -153.6092)
  line L498 (-60.7008, -153.6092) -> (-60.7008, -157.6092)
  line L499 (-60.7008, -157.6092) -> (-42.4786, -157.6092)
  line L500 (-42.4786, -157.6092) -> (-42.4786, -137.6092)
  line L501 (-42.4786, -137.6092) -> (-34.4786, -137.6092)
  line L502 (-34.4786, -137.6092) -> (-34.4786, -157.6092)
  line L503 (-34.4786, -157.6092) -> (-16.2564, -157.6092)
  line L504 (-16.2564, -157.6092) -> (-16.2564, -153.6092)
  line L505 (-16.2564, -153.6092) -> (5.9658, -153.6092)
  line L506 (5.9658, -153.6092) -> (5.9658, -157.6092)
  line L507 (5.9658, -157.6092) -> (24.1881, -157.6092)
  line L508 (24.1881, -157.6092) -> (24.1881, -137.6092)
  line L509 (24.1881, -137.6092) -> (32.1881, -137.6092)
  line L510 (32.1881, -137.6092) -> (32.1881, -157.6092)
  line L511 (32.1881, -157.6092) -> (50.4103, -157.6092)
  line L512 (50.4103, -157.6092) -> (50.4103, -153.6092)
  line L513 (50.4103, -153.6092) -> (72.6325, -153.6092)
  line L514 (72.6325, -153.6092) -> (72.6325, -157.6092)
  line L515 (72.6325, -157.6092) -> (90.8547, -157.6092)
  line L516 (90.8547, -157.6092) -> (90.8547, -145.6092)
  line L517 (90.8547, -145.6092) -> (94.8547, -145.6092)
  line L518 (94.8547, -145.6092) -> (94.8547, -129.6092)
  line L519 (94.8547, -129.6092) -> (90.8547, -129.6092)
  line L520 (90.8547, -129.6092) -> (90.8547, -117.6092)
  line L521 (90.8547, -117.6092) -> (-101.1453, -117.6092)
  line L522 (-101.1453, -117.6092) -> (-101.1453, -129.6092)
  line L523 (-101.1453, -129.6092) -> (-105.1453, -129.6092)
  line L524 (-105.1453, -129.6092) -> (-105.1453, -145.6092)
  line L525 (-105.1453, -145.6092) -> (-101.1453, -145.6092)
  line L526 (-101.1453, -145.6092) -> (-101.1453, -157.6092)
  line L527 (-101.1453, -157.6092) -> (-82.923, -157.6092)
  line L528 (-62.8232, -174.3606) -> (-62.8232, -178.3606)
  line L529 (-62.8232, -178.3606) -> (-85.0454, -178.3606)
  line L530 (-85.0454, -178.3606) -> (-85.0454, -174.3606)
  line L531 (-85.0454, -174.3606) -> (-103.2676, -174.3606)
  line L532 (-103.2676, -174.3606) -> (-103.2676, -186.3606)
  line L533 (-103.2676, -186.3606) -> (-107.2676, -186.3606)
  line L534 (-107.2676, -186.3606) -> (-107.2676, -202.3606)
  line L535 (-107.2676, -202.3606) -> (-103.2676, -202.3606)
  line L536 (-103.2676, -202.3606) -> (-103.2676, -214.3606)
  line L537 (-103.2676, -214.3606) -> (-44.601, -214.3606)
  line L538 (-44.601, -214.3606) -> (-44.601, -194.3606)
  line L539 (-44.601, -194.3606) -> (-36.601, -194.3606)
  line L540 (-36.601, -194.3606) -> (-36.601, -214.3606)
  line L541 (-36.601, -214.3606) -> (22.0657, -214.3606)
  line L542 (22.0657, -214.3606) -> (22.0657, -194.3606)
  line L543 (22.0657, -194.3606) -> (30.0657, -194.3606)
  line L544 (30.0657, -194.3606) -> (30.0657, -214.3606)
  line L545 (30.0657, -214.3606) -> (88.7324, -214.3606)
  line L546 (88.7324, -214.3606) -> (88.7324, -202.3606)
  line L547 (88.7324, -202.3606) -> (92.7324, -202.3606)
  line L548 (92.7324, -202.3606) -> (92.7324, -186.3606)
  line L549 (92.7324, -186.3606) -> (88.7324, -186.3606)
  line L550 (88.7324, -186.3606) -> (88.7324, -174.3606)
  line L551 (88.7324, -174.3606) -> (70.5101, -174.3606)
  line L552 (70.5101, -174.3606) -> (70.5101, -178.3606)
  line L553 (70.5101, -178.3606) -> (48.2879, -178.3606)
  line L554 (48.2879, -178.3606) -> (48.2879, -174.3606)
  line L555 (48.2879, -174.3606) -> (3.8435, -174.3606)
  line L556 (3.8435, -174.3606) -> (3.8435, -178.3606)
  line L557 (3.8435, -178.3606) -> (-18.3787, -178.3606)
  line L558 (-18.3787, -178.3606) -> (-18.3787, -174.3606)
  line L559 (-18.3787, -174.3606) -> (-62.8232, -174.3606)
  line L560 (-64.0936, -234.0705) -> (-64.0936, -238.0705)
  line L561 (-64.0936, -238.0705) -> (-86.3158, -238.0705)
  line L562 (-86.3158, -238.0705) -> (-86.3158, -234.0705)
  line L563 (-86.3158, -234.0705) -> (-104.5381, -234.0705)
  line L564 (-104.5381, -234.0705) -> (-104.5381, -246.0705)
  line L565 (-104.5381, -246.0705) -> (-108.5381, -246.0705)
  line L566 (-108.5381, -246.0705) -> (-108.5381, -262.0705)
  line L567 (-108.5381, -262.0705) -> (-104.5381, -262.0705)
  line L568 (-104.5381, -262.0705) -> (-104.5381, -274.0705)
  line L569 (-104.5381, -274.0705) -> (-45.8714, -274.0705)
  line L570 (-45.8714, -274.0705) -> (-45.8714, -254.0705)
  line L571 (-45.8714, -254.0705) -> (-37.8714, -254.0705)
  line L572 (-37.8714, -254.0705) -> (-37.8714, -274.0705)
  line L573 (-37.8714, -274.0705) -> (20.7953, -274.0705)
  line L574 (20.7953, -274.0705) -> (20.7953, -254.0705)
  line L575 (20.7953, -254.0705) -> (28.7953, -254.0705)
  line L576 (28.7953, -254.0705) -> (28.7953, -274.0705)
  line L577 (28.7953, -274.0705) -> (87.4619, -274.0705)
  line L578 (87.4619, -274.0705) -> (87.4619, -262.0705)
  line L579 (87.4619, -262.0705) -> (91.4619, -262.0705)
  line L580 (91.4619, -262.0705) -> (91.4619, -246.0705)
  line L581 (91.4619, -246.0705) -> (87.4619, -246.0705)
  line L582 (87.4619, -246.0705) -> (87.4619, -234.0705)
  line L583 (87.4619, -234.0705) -> (69.2397, -234.0705)
  line L584 (69.2397, -234.0705) -> (69.2397, -238.0705)
  line L585 (69.2397, -238.0705) -> (47.0175, -238.0705)
  line L586 (47.0175, -238.0705) -> (47.0175, -234.0705)
  line L587 (47.0175, -234.0705) -> (2.5731, -234.0705)
  line L588 (2.5731, -234.0705) -> (2.5731, -238.0705)
  line L589 (2.5731, -238.0705) -> (-19.6492, -238.0705)
  line L590 (-19.6492, -238.0705) -> (-19.6492, -234.0705)
  line L591 (-19.6492, -234.0705) -> (-64.0936, -234.0705)
  line L592 (150.9554, 76.4807) -> (140.9023, 86.5338)
  line L593 (140.9023, 86.5338) -> (145.5456, 91.1771)
  line L594 (145.5456, 91.1771) -> (155.5987, 81.124)
  line L595 (155.5987, 81.124) -> (165.6519, 91.1771)
  line L596 (165.6519, 91.1771) -> (170.2952, 86.5338)
  line L597 (170.2952, 86.5338) -> (160.2421, 76.4807)
  line L598 (160.2421, 76.4807) -> (170.2952, 66.4276)
  line L599 (170.2952, 66.4276) -> (165.6519, 61.7842)
  line L600 (165.6519, 61.7842) -> (155.5987, 71.8373)
  line L601 (155.5987, 71.8373) -> (145.5456, 61.7842)
  line L602 (145.5456, 61.7842) -> (140.9023, 66.4276)
  line L603 (140.9023, 66.4276) -> (150.9554, 76.4807)
  line L604 (164.858, 43.6473) -> (164.858, 48.1473)
  line L605 (164.858, 48.1473) -> (183.9321, 48.1473)
  line L606 (183.9321, 48.1473) -> (183.9321, 67.2214)
  line L607 (183.9321, 67.2214) -> (188.4321, 67.2214)
  line L608 (188.4321, 67.2214) -> (188.4321, 85.7399)
  line L609 (188.4321, 85.7399) -> (183.9321, 85.7399)
  line L610 (183.9321, 85.7399) -> (183.9321, 104.814)
  line L611 (183.9321, 104.814) -> (164.858, 104.814)
  line L612 (164.858, 104.814) -> (164.858, 109.314)
  line L613 (164.858, 109.314) -> (146.3395, 109.314)
  line L614 (146.3395, 109.314) -> (146.3395, 104.814)
  line L615 (146.3395, 104.814) -> (127.2654, 104.814)
  line L616 (127.2654, 104.814) -> (127.2654, 85.7399)
  line L617 (127.2654, 85.7399) -> (122.7654, 85.7399)
  line L618 (122.7654, 85.7399) -> (122.7654, 67.2214)
  line L619 (122.7654, 67.2214) -> (127.2654, 67.2214)
  line L620 (127.2654, 67.2214) -> (127.2654, 48.1473)
  line L621 (127.2654, 48.1473) -> (146.3395, 48.1473)
  line L622 (146.3395, 48.1473) -> (146.3395, 43.6473)
  line L623 (146.3395, 43.6473) -> (164.858, 43.6473)
  line L624 (75.0972, 74.6043) -> (65.0441, 64.5512)
  line L625 (65.0441, 64.5512) -> (60.4007, 69.1945)
  line L626 (60.4007, 69.1945) -> (70.4538, 79.2476)
  line L627 (70.4538, 79.2476) -> (60.4007, 89.3008)
  line L628 (60.4007, 89.3008) -> (65.0441, 93.9441)
  line L629 (65.0441, 93.9441) -> (75.0972, 83.891)
  line L630 (75.0972, 83.891) -> (85.1503, 93.9441)
  line L631 (85.1503, 93.9441) -> (89.7936, 89.3008)
  line L632 (89.7936, 89.3008) -> (79.7405, 79.2476)
  line L633 (79.7405, 79.2476) -> (89.7936, 69.1945)
  line L634 (89.7936, 69.1945) -> (85.1503, 64.5512)
  line L635 (85.1503, 64.5512) -> (75.0972, 74.6043)
  line L636 (42.2638, 69.9884) -> (46.7638, 69.9884)
  line L637 (46.7638, 69.9884) -> (46.7638, 50.9143)
  line L638 (46.7638, 50.9143) -> (65.8379, 50.9143)
  line L639 (65.8379, 50.9143) -> (65.8379, 46.4143)
  line L640 (65.8379, 46.4143) -> (84.3564, 46.4143)
  line L641 (84.3564, 46.4143) -> (84.3564, 50.9143)
  line L642 (84.3564, 50.9143) -> (103.4305, 50.9143)
  line L643 (103.4305, 50.9143) -> (103.4305, 69.9884)
  line L644 (103.4305, 69.9884) -> (107.9305, 69.9884)
  line L645 (107.9305, 69.9884) -> (107.9305, 88.5069)
  line L646 (107.9305, 88.5069) -> (103.4305, 88.5069)
  line L647 (103.4305, 88.5069) -> (103.4305, 107.581)
  line L648 (103.4305, 107.581) -> (84.3564, 107.581)
  line L649 (84.3564, 107.581) -> (84.3564, 112.081)
  line L650 (84.3564, 112.081) -> (65.8379, 112.081)
  line L651 (65.8379, 112.081) -> (65.8379, 107.581)
  line L652 (65.8379, 107.581) -> (46.7638, 107.581)
  line L653 (46.7638, 107.581) -> (46.7638, 88.5069)
  line L654 (46.7638, 88.5069) -> (42.2638, 88.5069)
  line L655 (42.2638, 88.5069) -> (42.2638, 69.9884)
  point P0 (156.6136, 48.0298)
  point P1 (175.9259, 62.6667)
equation "haed_rammi = 40 mm"
equation "lengd_rammi = 200 mm"
equation "d3 = haed_rammi"
equation "d4 = lengd_rammi"
equation "efni = 4 mm"
equation "d6 = þykkt"
equation "lfingur = 3"
equation "bfingur = 3"
equation "hfingur = 2"
equation "breidd_rammi = 200 mm"
equation "hfingur_br = haed_rammi / ( ( hfingur * 2 ) + 1 )"
equation "d13 = hfingur_br"
equation "d14 = hfingur_br"
equation "d15 = -þykkt"
equation "d17 = hfingur"
equation "d19 = -( haed_rammi - hfingur_br * 3 )"
equation "d21 = breidd_rammi"
equation "d22 = haed_rammi"
equation "d23 = þykkt"
equation "d26 = -þykkt"
equation "d32 = -þykkt"
equation "topp_fingur = 3"
equation "bfingur_toppur = breidd_rammi / ( 3 * topp_fingur )"
equation "lfingur_toppur = lengd_rammi / ( 3 * topp_fingur )"
equation "got_hlidar = 2"
equation "lengd_a_gotum = 2 * efni"
equation "got_fra_brun = ( haed_rammi - 2 * hfingur_br ) / 2"
equation "haed_a_gotum = 2 * hfingur_br"
equation "d53 = lengd_a_gotum"
equation "d54 = haed_a_gotum"
equation "d55 = got_fra_brun"
equation "got_fra_brun_breidd = ( breidd_rammi / 3 - efni )"
equation "d57 = got_fra_brun_lengd"
equation "d58 = -efni"
equation "d64 = got_hlidar"
equation "d66 = -( got_fra_brun_lengd + efni )"
equation "d68 = lengd_a_gotum"
equation "d69 = haed_a_gotum"
equation "d70 = got_fra_brun_breidd"
equation "d71 = got_fra_brun"
equation "d72 = -efni"
equation "d74 = got_hlidar"
equation "d76 = -( got_fra_brun_breidd + efni )"
equation "d78 = lengd_a_gotum"
equation "d80 = got_fra_brun_lengd"
equation "d82 = -efni"
equation "d84 = got_hlidar"
equation "d86 = -( got_fra_brun_lengd + efni )"
equation "d92 = lengd_a_gotum"
equation "d93 = got_fra_brun"
equation "d94 = haed_a_gotum"
equation "d95 = got_fra_brun_breidd"
equation "d96 = -efni"
equation "d98 = got_hlidar"
equation "d100 = -( got_fra_brun_breidd + efni )"
equation "got_fra_brun_lengd = lengd_rammi / 3 - efni"
equation "d103 = efni"
equation "d104 = got_fra_brun_breidd"
equation "d105 = lengd_rammi"
equation "d113 = haed_rammi"
equation "d114 = efni"
equation "d115 = got_fra_brun_breidd + efni"
equation "d116 = -lengd_rammi"
equation "d124 = efni"
equation "d125 = haed_rammi"
equation "d126 = 2 * got_fra_brun_breidd + 1 * efni"
equation "d127 = lengd_rammi"
equation "d129 = haed_rammi"
equation "d130 = efni"
equation "d131 = got_fra_brun_breidd"
equation "d132 = lengd_rammi"
equation "d134 = haed_rammi"
equation "d148 = haed_rammi / 2"
equation "d149 = 2 * efni"
equation "d151 = -2 * efni"
equation "d153 = got_hlidar"
equation "d155 = -( got_fra_brun_lengd + efni )"
equation "d157 = 2 * efni"
equation "d158 = haed_rammi / 2"
equation "d159 = got_fra_brun_lengd"
equation "d160 = -2 * efni"
equation "d162 = got_hlidar"
equation "d164 = -( got_fra_brun_lengd + efni )"
equation "d166 = efni"
equation "d167 = haed_rammi"
equation "d168 = got_fra_brun_lengd"
equation "d169 = -breidd_rammi"
equation "d171 = efni"
equation "d172 = haed_rammi"
equation "d173 = got_fra_brun_lengd + efni"
equation "d174 = -( breidd_rammi )"
equation "d178 = haed_a_gotum"
equation "d179 = got_fra_brun"
equation "d180 = haed_rammi"
equation "d181 = efni"
equation "d182 = got_fra_brun_lengd"
equation "d183 = breidd_rammi"
equation "d185 = haed_rammi"
equation "d186 = efni"
equation "d187 = got_fra_brun_lengd + efni"
equation "d188 = breidd_rammi"
equation "pusl_fingur_l = lfingur_toppur - lfingur_toppur / 6"
equation "pusl_fingurb = bfingur_toppur - lfingur_toppur / 6"
equation "d194 = efni"
equation "lengd_brun_toppur = lengd_rammi / ( 3 * topp_fingur )"
equation "d196 = lfingur_toppur"
equation "d197 = lengd_brun_toppur"
equation "d199 = got_fra_brun_lengd - efni"
equation "d200 = haed_rammi / 2"
equation "d201 = 2 * efni"
equation "d202 = got_fra_brun_lengd - efni"
equation "d203 = -efni"
equation "d207 = got_fra_brun_lengd + efni"
equation "d209 = -efni"
equation "d211 = topp_fingur"
equation "d213 = -( 2 * got_fra_brun_lengd + 2 * efni )"
equation "d215 = efni"
equation "d216 = bfingur_toppur"
equation "d217 = breidd_brun_toppur"
equation "breidd_brun_toppur = ( breidd_rammi / ( 3 * topp_fingur ) )"
equation "d219 = -efni"
equation "d221 = topp_fingur"
equation "d223 = got_fra_brun_breidd * 2 + 2 * efni"
equation "d225 = efni"
equation "d226 = lfingur_toppur"
equation "d227 = lengd_brun_toppur"
equation "d228 = -efni"
equation "d230 = topp_fingur"
equation "d232 = -( got_fra_brun_lengd * 2 + 2 * efni )"
equation "d234 = efni"
equation "d235 = bfingur_toppur"
equation "d236 = breidd_brun_toppur"
equation "d237 = -efni"
equation "d239 = topp_fingur"
equation "d241 = -( got_fra_brun_breidd * 2 + 2 * efni )"
equation "d245 = 2 * efni"
equation "d246 = bfingur_toppur"
equation "d247 = breidd_brun_toppur"
equation "d248 = -efni"
equation "d250 = topp_fingur"
equation "d252 = -( got_fra_brun_breidd * 2 + 2 * efni )"
equation "d254 = 2 * efni"
equation "d255 = bfingur_toppur"
equation "d256 = breidd_brun_toppur"
equation "d257 = -efni"
equation "d259 = topp_fingur"
equation "d261 = -( got_fra_brun_breidd * 2 + 2 * efni )"
equation "d263 = 2 * efni"
equation "d264 = lfingur_toppur"
equation "d265 = lengd_brun_toppur"
equation "d266 = -efni"
equation "d268 = topp_fingur"
equation "d270 = -( 2 * got_fra_brun_lengd + 2 * efni )"
equation "d272 = 2 * efni"
equation "d273 = lfingur_toppur"
equation "d274 = lengd_brun_toppur"
equation "d275 = -efni"
equation "d277 = topp_fingur"
equation "d279 = 2 * got_fra_brun_lengd + 2 * efni"
equation "lengd_fra_fingri_ad_brun_pusl = lengd_brun_toppur - efni"
equation "breidd_fra_fingri_ad_brun_pusl = breidd_brun_toppur - efni"
equation "d295 = breidd_rammi"
equation "d296 = lengd_rammi"
equation "d297 = -efni"
equation "d299 = bil_milli_pusla"
equation "bil_milli_pusla = 1 mm"
equation "d301 = 2 * efni"
equation "d302 = ( lfingur_toppur - pusl_fingur_l ) / 2"
equation "d303 = ( lengd_brun_toppur - pusl_fingur_l ) / 2"
equation "d304 = 2 * efni"
equation "d305 = efni - bil_milli_pusla / 2"
equation "d306 = lfingur_toppur"